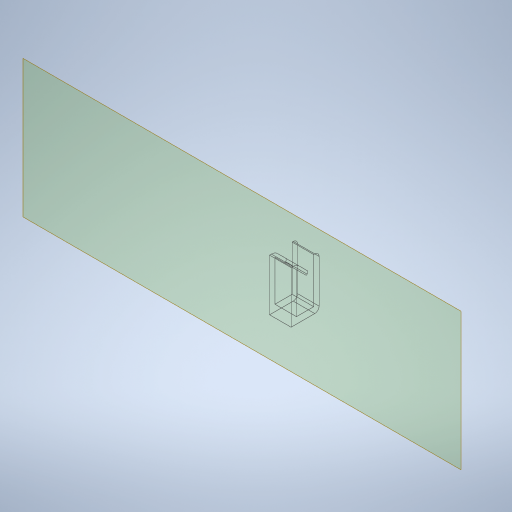
# Autodesk Inventor part: cable-clip
Saved by Autodesk Inventor 2024 (Build 280153000, 153)
## iProperties
Created: 2024-04-22
Part Number: cable-clip
Material: Generic
Document SubType Name: Modeling
Designer: MaartenGeorgesBuelen
Density: 1 g/cm^3
Appearance: Default
Author: MaartenGeorgesBuelen
## iProperties of the stored document cable-clip_3DPrint.ipt
Created: 2024-04-22
Part Number: cable-clip_3DPrint
Material: Generic
Document SubType Name: Modeling
Designer: MaartenGeorgesBuelen
Density: 1 g/cm^3
Appearance: Default
Author: MaartenGeorgesBuelen
Autodesk Inventor part; units mm, degrees
ref_plane "YZ Plane" through (0, 0, 0) normal (1, 0, 0) x (0, 1, 0)
ref_plane "XZ Plane" through (0, 0, 0) normal (0, 1, 0) x (-1, 0, 0)
ref_plane "XY Plane" through (0, 0, 0) normal (0, 0, 1) x (1, 0, 0)
ref_plane "Work Plane1" through (150, 0, -50) normal (0, 0, -1) x (-1, 0, 0)
sketch "Sketch1" plane through (150, 0, -50) normal (0, 0, -1) x (-1, 0, 0)
  line L0 (-107, 15) -> (222, 15)
  line L1 (44.694, 5) -> (34.694, 5)
  line L2 (34.694, 5) -> (34.694, 25)
  line L3 (34.694, 25) -> (44.694, 25)
  line L4 (44.694, 25) -> (44.694, 5)
  line L5 (44.694, 5) -> (34.694, 25) construction
  line L6 (34.694, 5) -> (44.694, 25) construction
  line L7 (34.694, 5) -> (44.694, 5)
  line L8 (44.694, 5) -> (44.694, 1)
  line L9 (44.694, 1) -> (34.694, 1)
  line L10 (34.694, 1) -> (34.694, 5)
  point P0 (150, 0)
  point P1 (39.694, 15)
  dimension "d0" = 20
  dimension "d1" = 10
  dimension "d2" = 177.306
  dimension "d3" = 4
  constraints: 22 end point, 4 parallel, 3 horizontal, 2 midpoint, 2 perpendicular, 1 point on line, 2 other
  measures "d0" distance of L1.end L2.end
  measures "d1" distance between parallel lines of L2 L4
  measures "d2" distance from line of L0.end L4
  measures "d3" distance of L7.end L8.end
extrude "Extrusion1" add sketch "Sketch1" along normal blind 2.5
sketch "Sketch2" plane through (150, 0, -52.5) normal (0, 0, -1) x (-1, 0, 0)
  line L0 (34.694, 25) -> (34.694, 1) projected
  line L1 (34.694, 1) -> (44.694, 1) projected
  line L2 (44.694, 1) -> (44.694, 25) projected
  line L3 (44.694, 25) -> (34.694, 25) projected
  line L4 (34.694, 1) -> (44.694, 1)
  line L5 (44.694, 1) -> (44.694, 4)
  line L6 (44.694, 4) -> (34.694, 4)
  line L7 (34.694, 4) -> (34.694, 1)
  point P0 (150, 0)
  dimension "d6" = 3
  constraints: 8 end point, 2 parallel, 1 horizontal, 1 perpendicular, 1 point on line
  measures "d6" distance of L5.end L4.end
extrude "Extrusion2" add sketch "Sketch2" along normal blind 8 contours L6 L2 L1 L0
sketch "Sketch3" plane through (150, 0, -60.5) normal (0, 0, -1) x (-1, 0, 0)
  line L0 (34.694, 4) -> (34.694, 1) projected
  line L1 (34.694, 1) -> (44.694, 1) projected
  line L2 (44.694, 1) -> (44.694, 4) projected
  line L3 (44.694, 4) -> (34.694, 4) projected
  line L4 (-107, 15) -> (222, 15)
  line L5 (34.694, 4) -> (44.694, 4) projected
  line L6 (44.694, 4) -> (44.694, 25) projected
  line L7 (44.694, 25) -> (34.694, 25) projected
  line L8 (34.694, 25) -> (34.694, 4) projected
  line L9 (34.694, 25) -> (44.694, 25)
  line L10 (44.694, 25) -> (44.694, 1)
  line L11 (44.694, 1) -> (34.694, 1)
  line L12 (34.694, 1) -> (34.694, 25)
  point P0 (150, 0)
  constraints: 10 end point, 2 horizontal, 2 parallel, 1 perpendicular, 2 other
extrude "Extrusion3" add sketch "Sketch3" along normal blind 2.5
sketch "Sketch4" plane through (115.306, 1, -50) normal (1, 0, 0) x (0, 0, -1)
  line L0 (2.5, 3) -> (2.5, 24) projected
  line L1 (2.5, 24) -> (8.1569, 18.3431)
  line L2 (2.5, 24) -> (10.5, 24) construction
  line L3 (8.1569, 18.3431) -> (7.0962, 17.2825)
  line L4 (7.0962, 17.2825) -> (2.5, 21.8787)
  point P0 (-50, -1)
  dimension "d11" = 8
  dimension "d12" = 45
  dimension "d13" = 1.5
  constraints: 8 end point, 2 perpendicular, 1 equal length, 1 horizontal, 1 point on line
  measures "d11" distance of L0.end L1.end
  measures "d12" angle of L1 L2
  measures "d13" distance of L1.end L3.end
extrude "Extrusion4" add sketch "Sketch4" against normal up to surface (10 mm away)
fillet "Fillet1" radius 2 2 edges at (110.306, 25, -63) (110.306, 1, -63)
fillet "Fillet2" radius 4 1 edges at (110.306, 25, -52.5)
fillet "Fillet3" radius 1 1 edges at (110.306, 19.3431, -58.1569)
body "Solid1"
